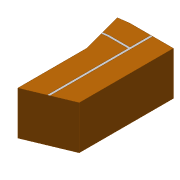
# Autodesk Inventor part: Hill 3
Saved by Autodesk Inventor 2015 SP1 (Build 190203100, 203)
## iProperties
Created: 2015-08-24
Part Number: Hill 3
Material: 一般
Document SubType Name: Modeling
Designer: nobuhiro
Density: 1 g/cm^3
Appearance: オレンジ
Author: nobuhiro
Autodesk Inventor part; units mm, degrees
ref_plane "YZ Plane" through (0, 0, 0) normal (1, 0, 0) x (0, 1, 0)
ref_plane "XZ Plane" through (0, 0, 0) normal (0, 1, 0) x (-1, 0, 0)
ref_plane "XY Plane" through (0, 0, 0) normal (0, 0, 1) x (1, 0, 0)
sketch "スケッチ1" plane through (0, 0, 0) normal (0, 0, 1) x (1, 0, 0)
  line L0 (-300, 0) -> (300, 0)
  line L1 (300, 0) -> (300, -1301.4719)
  line L2 (300, -1301.4719) -> (-300, -1301.4719)
  line L3 (-300, -1301.4719) -> (-300, 0)
  line L4 (300, -1301.4719) -> (-300, -1550)
  line L5 (-300, -1550) -> (-300, -1301.4719)
  line L6 (-300, -600) -> (-455.2914, -20.4445)
  line L7 (-455.2914, -20.4445) -> (-300, 0)
  point P0 (0, 0)
  point P1 (0, 0)
  dimension "d18" = 600
  dimension "d27" = 67.5
  dimension "d28" = 1550
  dimension "d29" = 600
  dimension "d30" = 600
  dimension "d31" = 15
  constraints: 16 end point, 2 coincident, 2 parallel, 1 collinear, 1 horizontal, 1 midpoint, 1 perpendicular, 1 point on line
  measures "d18" distance between parallel lines of L3 L1
  measures "d27" angle of L5 L4
  measures "d28" distance from line of L0 L4.end
  measures "d29" distance of L6.start L6.end
  measures "d30" distance from line of L6.start L0
  measures "d31" angle of L6 L3
extrude "押し出し1" add sketch "スケッチ1" along normal blind 600
sketch "スケッチ3" plane through (0, 0, 600) normal (0, 0, 1) x (1, 0, 0)
  line L0 (300, 0) -> (-300, 0) projected
  line L1 (15, 0) -> (-15, 0)
  line L2 (-15, 0) -> (-15, -1431.9491)
  line L3 (15, -1419.5227) -> (15, 0)
  line L4 (-15, -285) -> (-300, -285)
  line L5 (-373.7634, -324.7111) -> (-300, -315)
  line L6 (-15, -315) -> (-15, -285)
  line L7 (-15, -1431.9491) -> (15, -1419.5227)
  line L8 (-373.7634, -324.7111) -> (-381.528, -295.7334)
  line L9 (-300, -1550) -> (300, -1301.4719) projected
  line L10 (-455.2914, -20.4445) -> (-300, -600) projected
  line L11 (-300, 0) -> (-455.2914, -20.4445) projected
  line L12 (-300, -600) -> (-300, 0)
  line L13 (-300, -285) -> (-381.528, -295.7334)
  line L14 (-300, -315) -> (-15, -315)
  point P0 (0, 0)
  point P1 (0, 0)
  point P2 (0, 0)
  dimension "d23" = 30
  dimension "d24" = 285
  dimension "d33" = 30
  constraints: 22 end point, 8 point on line, 4 parallel, 2 horizontal, 2 midpoint, 1 coincident, 1 perpendicular, 1 vertical
  measures "d23" distance between parallel lines of L2 L3
  measures "d24" distance between parallel lines of L0 L4
  measures "d33" distance between parallel lines of L14 L4
extrude "押し出し3" add sketch "スケッチ3" along normal blind 0.1 contours L3 L7 L2 L0 | L2 L14 L12 L4 | L12 L5 L8 L13
